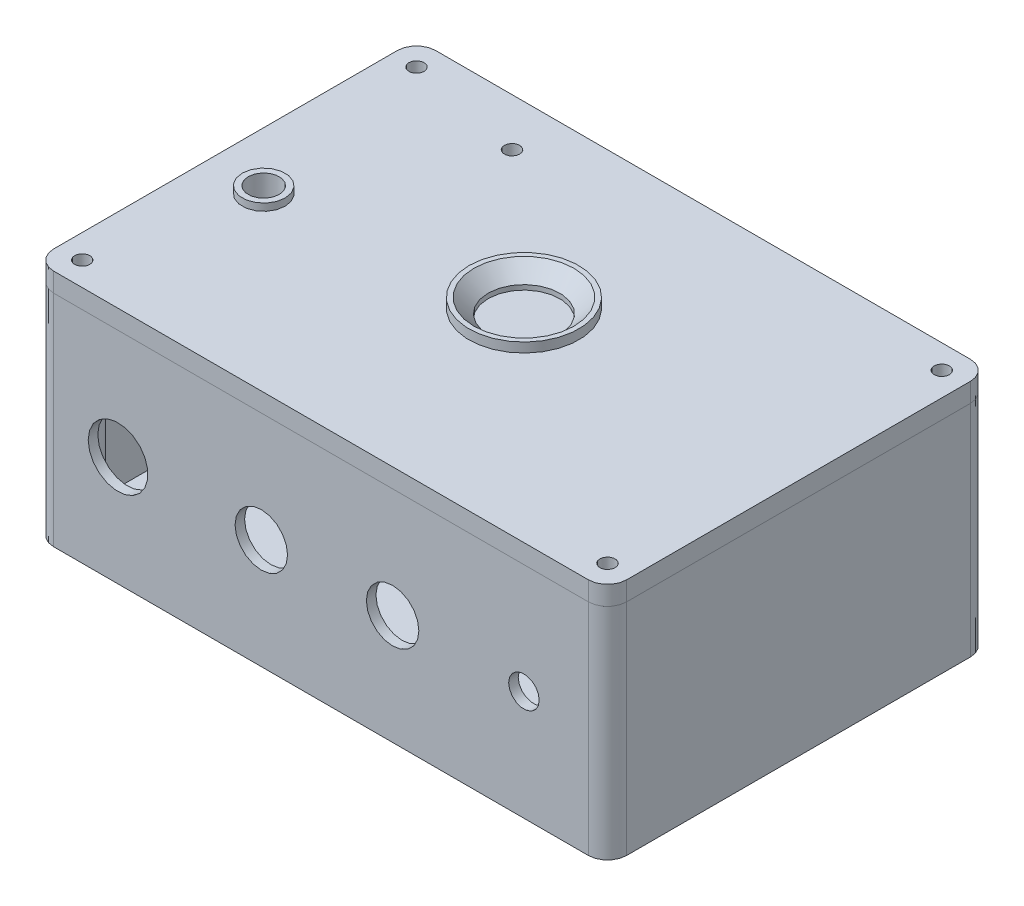
GridUp-Kutu (Autodesk Fusion 360 design; units mm, degrees)
part number: 2026-09-14-07-36-03-763
Autodesk Fusion 360 part; units mm, degrees
sketch "Çizim1" plane through (0, 0, 0) normal (0, 0, 1) x (1, 0, 0)
  line L0 (0, 0) -> (120, 0)
  line L1 (120, 0) -> (120, 80)
  line L2 (120, 80) -> (0, 80)
  line L3 (0, 80) -> (0, 0)
extrude "Ekstrüzyon1" add sketch "Çizim1" along normal blind 46 makes body 1
fillet "Radyus1" radius 4 4 edges at (0, 80, 23) (120, 80, 23) (120, 0, 23) (0, 0, 23) on bodies 1
shell "Kabuk1" thickness 2 removed faces 1 at (78.6667, 26.6667, 46) on bodies 1
sketch "Çizim2" plane through (0, 0, 0) normal (0, 0, 1) x (1, 0, 0)
  circle A0 centre (5, 5) radius 3.5
  circle A1 centre (115, 5) radius 3.5
  circle A2 centre (5, 75) radius 3.5
  circle A3 centre (115, 75) radius 3.5
extrude "Ekstrüzyon2" add sketch "Çizim2" along normal blind 46 bodies 1
ref_plane "WorkPlane1" through (0, 0, 46) normal (0, 0, 1) x (1, 0, 0)
sketch "Çizim3" plane through (0, 0, 46) normal (0, 0, 1) x (1, 0, 0)
  line L0 (0, 0) -> (120, 0)
  line L1 (120, 0) -> (120, 80)
  line L2 (120, 80) -> (0, 80)
  line L3 (0, 80) -> (0, 0)
extrude "Ekstrüzyon3" add sketch "Çizim3" along normal blind 4 separate body makes body 2
fillet "Radyus2" radius 4 4 edges at (0, 80, 48) (120, 80, 48) (120, 0, 48) (0, 0, 48) on bodies 2
ref_plane "WorkPlane2" through (0, 0, 50) normal (0, 0, 1) x (1, 0, 0)
sketch "Çizim4" plane through (0, 0, 50) normal (0, 0, 1) x (1, 0, 0)
  circle A0 centre (60, 42.5) radius 11.5
extrude "Ekstrüzyon4" add sketch "Çizim4" along normal blind 2 bodies 2
sketch "Çizim5" plane through (0, 0, 50) normal (0, 0, 1) x (1, 0, 0)
  circle A0 centre (60, 42.5) radius 7.5
extrude "Ekstrüzyon5" cut sketch "Çizim5" along normal mid plane 16 bodies 2
chamfer "Pah1" distance 3 angle 45 1 edges at (53.0075, 45.2121, 52) tangent chain off on bodies 2
sketch "Çizim6" plane through (0, 0, 50) normal (0, 0, 1) x (1, 0, 0)
  circle A0 centre (12, 36) radius 4.5
extrude "Ekstrüzyon6" add sketch "Çizim6" along normal blind 1.5 bodies 2
sketch "Çizim7" plane through (0, 0, 50) normal (0, 0, 1) x (1, 0, 0)
  circle A0 centre (12, 36) radius 3.25
extrude "Ekstrüzyon7" cut sketch "Çizim7" along normal mid plane 16 bodies 2
sketch "Çizim8" plane through (0, 0, 50) normal (0, 0, 1) x (1, 0, 0)
  circle A0 centre (30, 70) radius 1.6
extrude "Ekstrüzyon8" cut sketch "Çizim8" along normal mid plane 16 bodies 2
sketch "Çizim9" plane through (0, 0, 50) normal (0, 0, 1) x (1, 0, 0)
  circle A0 centre (5, 5) radius 1.6
  circle A1 centre (115, 5) radius 1.6
  circle A2 centre (5, 75) radius 1.6
  circle A3 centre (115, 75) radius 1.6
extrude "Ekstrüzyon9" cut sketch "Çizim9" along normal mid plane 16 bodies 2
sketch "Çizim10" plane through (0, 0, 50) normal (0, 0, 1) x (1, 0, 0)
  circle A0 centre (5, 5) radius 1.25
  circle A1 centre (115, 5) radius 1.25
  circle A2 centre (5, 75) radius 1.25
  circle A3 centre (115, 75) radius 1.25
extrude "Ekstrüzyon10" cut sketch "Çizim10" against normal blind 16 bodies 1
ref_plane "WorkPlane3" through (0, 0, 47.5) normal (0, 0, 1) x (1, 0, 0)
sketch "Çizim11" plane through (0, 0, 47.5) normal (0, 0, 1) x (1, 0, 0)
  circle A0 centre (60, 42.5) radius 7.5
extrude "Ekstrüzyon11" add sketch "Çizim11" along normal mid plane 1 separate body makes body 3
sketch "Çizim12" plane through (0, 0, 0) normal (0, 1, 0) x (1, 0, 0)
  circle A0 centre (17.5, -23) radius 6.25
  circle A1 centre (47.5, -23) radius 5.5
  circle A2 centre (75, -23) radius 5.5
  circle A3 centre (102.5, -23) radius 3.2
extrude "Ekstrüzyon12" cut sketch "Çizim12" along normal mid plane 6 bodies 1
sketch "Çizim13" plane through (0, 0, 0) normal (0, 0, 1) x (1, 0, 0)
  line L0 (12.75, 42.5) -> (22.25, 42.5)
  arc A0 (22.25, 42.5) -> (22.25, 48) centre (22.25, 45.25) ccw
  line L1 (22.25, 48) -> (12.75, 48)
  arc A1 (12.75, 48) -> (12.75, 42.5) centre (12.75, 45.25) ccw
  line L2 (97.75, 42.5) -> (107.25, 42.5)
  arc A2 (107.25, 42.5) -> (107.25, 48) centre (107.25, 45.25) ccw
  line L3 (107.25, 48) -> (97.75, 48)
  arc A3 (97.75, 48) -> (97.75, 42.5) centre (97.75, 45.25) ccw
extrude "Ekstrüzyon13" cut sketch "Çizim13" along normal mid plane 6 bodies 1
sketch "Çizim14" plane through (0, 0, 0) normal (0, 0, 1) x (1, 0, 0)
  circle A0 centre (7.5, 7.5) radius 3.5
  circle A1 centre (112.5, 7.5) radius 3.5
  circle A2 centre (7.5, 72.5) radius 3.5
  circle A3 centre (112.5, 72.5) radius 3.5
extrude "Ekstrüzyon14" cut sketch "Çizim14" along normal mid plane 2 bodies 1
sketch "Çizim15" plane through (0, 0, 0) normal (0, 0, 1) x (1, 0, 0)
  line L0 (42.5, 20) -> (77.5, 20)
  line L1 (77.5, 20) -> (77.5, 62)
  line L2 (77.5, 62) -> (42.5, 62)
  line L3 (42.5, 62) -> (42.5, 20)
extrude "Ekstrüzyon15" add sketch "Çizim15" against normal blind 5 separate body makes body 4
ref_plane "WorkPlane4" through (0, 0, -5) normal (0, 0, 1) x (1, 0, 0)
sketch "Çizim16" plane through (0, 0, -5) normal (0, 0, 1) x (1, 0, 0)
  line L0 (42.5, 23.25) -> (77.5, 23.25)
  line L1 (77.5, 23.25) -> (77.5, 58.75)
  line L2 (77.5, 58.75) -> (42.5, 58.75)
  line L3 (42.5, 58.75) -> (42.5, 23.25)
extrude "Ekstrüzyon16" cut sketch "Çizim16" along normal mid plane 6 bodies 4
equation "d29 = -( 16 mm )"
equation "d41 = -( 5 mm )"
named bodies: "Gövde", "Kapak", "IR pencere", "DIN klips"
